Autodesk Fusion 360 part; units mm, degrees
(part 3 of 7)
  spline S363 degree 3 poles (9.5018, -1.5566) (9.5018, -1.7848) (9.4886, -1.9954) (9.4755, -2.0349) knots 0 0 0 0 1 1 1 1
  spline S364 degree 3 poles (9.4755, -2.0349) (9.4404, -2.1271) (9.3701, -2.1227) (9.3701, -2.0305) knots 0 0 0 0 1 1 1 1
  spline S365 degree 3 poles (9.3701, -2.0305) (9.3701, -1.8989) (9.1902, -1.6444) (8.8699, -1.3152) knots 0 0 0 0 1 1 1 1
  spline S366 degree 3 poles (8.8699, -1.3152) (8.7031, -1.1485) (8.5539, -1.008) (8.5407, -1.008) knots 0 0 0 0 1 1 1 1
  spline S367 degree 3 poles (8.5407, -1.008) (8.4925, -1.008) (7.7201, -1.8067) (7.4173, -2.171) knots 0 0 0 0 1 1 1 1
  spline S368 degree 3 poles (7.4173, -2.171) (6.9653, -2.7195) (6.5264, -3.6894) (6.3158, -4.6153) knots 0 0 0 0 1 1 1 1
  spline S369 degree 3 poles (6.3158, -4.6153) (6.1446, -5.3745) (6.1841, -6.1469) (6.4431, -7.0509) knots 0 0 0 0 1 1 1 1
  spline S370 degree 3 poles (6.4431, -7.0509) (6.5923, -7.5731) (6.9302, -8.1392) (7.3646, -8.5913) knots 0 0 0 0 1 1 1 1
  spline S371 degree 3 poles (7.3646, -8.5913) (7.5358, -8.7624) (7.6543, -8.9072) (7.6367, -8.9072) knots 0 0 0 0 1 1 1 1
  spline S372 degree 3 poles (7.6367, -8.9072) (7.5446, -8.9072) (7.2286, -8.6395) (7.0004, -8.3674) knots 0 0 0 0 1 1 1 1
  spline S373 degree 3 poles (7.0004, -8.3674) (6.5791, -7.8672) (6.3114, -7.2659) (6.1183, -6.3839) knots 0 0 0 0 1 1 1 1
  spline S374 degree 3 poles (6.1183, -6.3839) (6.0569, -6.0942) (5.9779, -5.8748) (5.8638, -5.6817) knots 0 0 0 0 1 1 1 1
  spline S375 degree 3 poles (5.8638, -5.6817) (5.776, -5.5237) (5.6882, -5.4052) (5.6795, -5.414) knots 0 0 0 0 1 1 1 1
  spline S376 degree 3 poles (5.6795, -5.414) (5.6487, -5.4491) (5.6312, -5.278) (5.6312, -4.8699) knots 0 0 0 0 1 1 1 1
  spline S377 degree 3 poles (5.6312, -4.8699) (5.6268, -4.5407) (5.6444, -4.453) (5.7892, -4.1019) knots 0 0 0 0 1 1 1 1
  spline S378 degree 3 poles (5.7892, -4.1019) (5.9954, -3.5928) (6.3377, -2.9872) (6.7283, -2.4299) knots 0 0 0 0 1 1 1 1
  spline S379 degree 3 poles (6.7283, -2.4299) (7.0355, -1.991) (7.8254, -1.1441) (8.2511, -0.7974) knots 0 0 0 0 1 1 1 1
  spline S380 degree 3 poles (8.2511, -0.7974) (8.3696, -0.6965) (8.453, -0.6043) (8.4398, -0.5867) knots 0 0 0 0 1 1 1 1
  spline S381 degree 3 poles (8.4398, -0.5867) (8.4047, -0.5516) (7.7201, -0.5516) (7.5709, -0.5867) knots 0 0 0 0 1 1 1 1
  spline S382 degree 3 poles (7.5709, -0.5867) (7.448, -0.6131) (7.3602, -0.714) (7.3207, -0.8676) knots 0 0 0 0 1 1 1 1
  spline S383 degree 3 poles (7.3207, -0.8676) (7.2593, -1.1221) (7.2198, -0.9027) (7.2198, -0.2796) knots 0 0 0 0 1 1 1 1
  spline S384 degree 3 poles (7.2198, -0.2796) (7.2198, 0.3612) (7.2593, 0.5411) (7.3295, 0.2251) knots 0 0 0 0 1 1 1 1
  spline S385 degree 3 poles (7.3295, 0.2251) (7.3427, 0.1549) (7.4085, 0.0452) (7.4699, -0.0163) knots 0 0 0 0 1 1 1 1
  spline S386 degree 3 poles (7.4699, -0.0163) (7.5709, -0.1172) (7.6411, -0.1435) (7.8561, -0.1435) knots 0 0 0 0 1 1 1 1
  spline S387 degree 3 poles (7.8561, -0.1435) (7.8912, -0.1435) (8.4968, -0.1391) (9.2034, -0.1347) knots 0 0 0 0 1 1 1 1
  spline S388 degree 3 poles (9.2034, -0.1347) (10.6998, -0.1304) (10.6603, -0.1567) (9.8353, 0.3392) knots 0 0 0 0 1 1 1 1
  spline S389 degree 3 poles (9.8353, 0.3392) (9.2473, 0.6947) (7.1496, 2.0814) (7.0136, 2.2043) knots 0 0 0 0 1 1 1 1
  spline S390 degree 3 poles (7.0136, 2.2043) (6.9609, 2.2526) (6.8995, 2.2789) (6.8731, 2.2613) knots 0 0 0 0 1 1 1 1
  spline S391 degree 3 poles (6.8731, 2.2613) (6.838, 2.2438) (6.8249, 1.7084) (6.8249, 0.5762) knots 0 0 0 0 1 1 1 1
  spline S392 degree 3 poles (6.8249, 0.5762) (6.8249, -0.3366) (6.8117, -1.2626) (6.7985, -1.482) knots 0 0 0 0 1 1 1 1
  spline S393 degree 3 poles (6.7985, -1.482) (6.7722, -1.8462) (6.759, -1.8901) (6.6581, -1.9559) knots 0 0 0 0 1 1 1 1
  spline S394 degree 3 poles (6.6581, -1.9559) (6.5923, -1.9998) (6.5352, -2.0086) (6.5133, -1.9867) knots 0 0 0 0 1 1 1 1
  spline S395 degree 3 poles (6.5133, -1.9867) (6.4782, -1.9516) (6.4299, 3.0732) (6.465, 3.0732) knots 0 0 0 0 1 1 1 1
  spline S396 degree 3 poles (6.465, 3.0732) (6.4694, 3.0732) (6.5133, 3.0381) (6.5572, 2.9942) knots 0 0 0 0 1 1 1 1
  spline S397 degree 3 poles (6.5572, 2.9942) (6.6405, 2.9196) (7.0399, 2.6475) (8.431, 1.7216) knots 0 0 0 0 1 1 1 1
  spline S398 degree 3 poles (8.431, 1.7216) (8.8172, 1.4627) (9.2824, 1.1511) (9.4623, 1.0282) knots 0 0 0 0 1 1 1 1
  spline S399 degree 3 poles (9.4623, 1.0282) (9.7827, 0.8088) (10.3707, 0.4401) (10.4058, 0.4401) knots 0 0 0 0 1 1 1 1
  spline S400 degree 3 poles (10.4058, 0.4401) (10.4146, 0.4401) (10.4234, 0.7298) (10.4234, 1.0852) knots 0 0 0 0 1 1 1 1
  line L93 (10.4234, 1.0852) -> (10.419, 1.7347)
  line L94 (10.419, 1.7347) -> (10.1732, 1.8839)
  spline S401 degree 3 poles (10.1732, 1.8839) (9.9406, 2.0244) (9.9319, 2.0375) (10.0196, 2.077) knots 0 0 0 0 1 1 1 1
  spline S402 degree 3 poles (10.0196, 2.077) (10.0898, 2.1078) (10.1864, 2.0946) (10.3883, 2.02) knots 0 0 0 0 1 1 1 1
  spline S403 degree 3 poles (10.3883, 2.02) (10.5419, 1.9673) (10.6911, 1.9015) (10.7218, 1.8752) knots 0 0 0 0 1 1 1 1
  spline S404 degree 3 poles (10.7218, 1.8752) (10.7613, 1.8444) (10.7744, 1.6119) (10.7701, 0.9185) knots 0 0 0 0 1 1 1 1
  line L95 (10.7701, 0.9185) -> (10.7657, 0.0013)
  line L96 (10.7657, 0.0013) -> (10.6384, 0.0013)
  spline S405 degree 3 poles (10.6384, 0.0013) (10.5682, 0.0013) (10.5111, -0.0075) (10.5111, -0.0163) knots 0 0 0 0 1 1 1 1
  spline S406 degree 3 poles (10.5111, -0.0163) (10.5111, -0.0514) (10.8798, -0.3849) (11.1475, -0.5955) knots 0 0 0 0 1 1 1 1
  spline S407 degree 3 poles (11.1475, -0.5955) (11.5863, -0.9378) (12.0032, -1.3679) (12.0032, -1.482) knots 0 0 0 0 1 1 1 1
  spline S408 degree 3 poles (12.0032, -1.482) (12.0032, -1.5698) (11.9593, -1.5478) (11.6214, -1.2889) knots 0 0 0 0 1 1 1 1
  spline S409 degree 3 poles (11.2089, 5.9652) (11.1343, 5.9257) (11.1255, 5.9432) (11.1255, 6.1319) knots 0 0 0 0 1 1 1 1
  spline S410 degree 3 poles (11.1255, 6.1319) (11.1255, 6.404) (11.086, 6.5401) (11.0114, 6.5401) knots 0 0 0 0 1 1 1 1
  spline S411 degree 3 poles (11.0114, 6.5401) (10.9763, 6.5401) (10.8008, 6.4699) (10.6165, 6.3865) knots 0 0 0 0 1 1 1 1
  spline S412 degree 3 poles (10.6165, 6.3865) (10.4365, 6.3031) (10.2698, 6.2329) (10.2522, 6.2329) knots 0 0 0 0 1 1 1 1
  spline S413 degree 3 poles (10.2522, 6.2329) (10.2303, 6.2329) (10.0635, 6.1539) (9.8792, 6.0573) knots 0 0 0 0 1 1 1 1
  spline S414 degree 3 poles (9.8792, 6.0573) (9.6949, 5.9608) (9.5062, 5.8818) (9.4623, 5.8818) knots 0 0 0 0 1 1 1 1
  spline S415 degree 3 poles (9.4623, 5.8818) (9.414, 5.8818) (9.3658, 5.8643) (9.3482, 5.8423) knots 0 0 0 0 1 1 1 1
  spline S416 degree 3 poles (9.3482, 5.8423) (9.335, 5.8204) (9.1639, 5.737) (8.9664, 5.6624) knots 0 0 0 0 1 1 1 1
  spline S417 degree 3 poles (8.9664, 5.6624) (8.4661, 5.4693) (8.0799, 5.2674) (8.1238, 5.2235) knots 0 0 0 0 1 1 1 1
  spline S418 degree 3 poles (8.1238, 5.2235) (8.1458, 5.206) (8.2335, 5.1665) (8.3169, 5.1445) knots 0 0 0 0 1 1 1 1
  spline S419 degree 3 poles (8.3169, 5.1445) (8.4003, 5.1182) (8.7163, 5.0041) (9.0191, 4.89) knots 0 0 0 0 1 1 1 1
  spline S420 degree 3 poles (9.0191, 4.89) (9.3394, 4.7671) (9.6422, 4.6794) (9.7432, 4.6794) knots 0 0 0 0 1 1 1 1
  spline S421 degree 3 poles (9.7432, 4.6794) (9.9055, 4.6794) (10.8842, 5.0348) (11.029, 5.1489) knots 0 0 0 0 1 1 1 1
  spline S422 degree 3 poles (11.029, 5.1489) (11.0553, 5.1709) (11.0816, 5.2762) (11.0816, 5.3771) knots 0 0 0 0 1 1 1 1
  spline S423 degree 3 poles (11.0816, 5.3771) (11.0816, 5.5702) (11.1694, 5.6975) (11.2616, 5.6361) knots 0 0 0 0 1 1 1 1
  spline S424 degree 3 poles (11.2616, 5.6361) (11.3318, 5.5966) (11.2923, 3.8807) (11.2221, 3.8105) knots 0 0 0 0 1 1 1 1
  spline S425 degree 3 poles (11.2221, 3.8105) (11.1431, 3.7315) (11.0816, 3.9597) (11.0816, 4.3064) knots 0 0 0 0 1 1 1 1
  spline S426 degree 3 poles (11.0816, 4.3064) (11.0816, 4.7189) (11.1299, 4.7233) (9.9406, 4.2361) knots 0 0 0 0 1 1 1 1
  spline S427 degree 3 poles (9.9406, 4.2361) (9.6861, 4.1352) (9.2385, 3.9553) (8.9445, 3.8412) knots 0 0 0 0 1 1 1 1
  spline S428 degree 3 poles (8.9445, 3.8412) (8.6504, 3.7271) (8.374, 3.6086) (8.3301, 3.5779) knots 0 0 0 0 1 1 1 1
  spline S429 degree 3 poles (8.3301, 3.5779) (8.2599, 3.5252) (8.2686, 3.512) (8.4486, 3.4287) knots 0 0 0 0 1 1 1 1
  spline S430 degree 3 poles (8.4486, 3.4287) (8.9532, 3.2005) (10.8578, 2.4588) (10.95, 2.4588) knots 0 0 0 0 1 1 1 1
  spline S431 degree 3 poles (10.95, 2.4588) (11.007, 2.4588) (11.1255, 2.7441) (11.1255, 2.8845) knots 0 0 0 0 1 1 1 1
  spline S432 degree 3 poles (11.1255, 2.8845) (11.1255, 2.9503) (11.1475, 3.0381) (11.1694, 3.0732) knots 0 0 0 0 1 1 1 1
  spline S433 degree 3 poles (11.1694, 3.0732) (11.2659, 3.218) (11.2967, 2.9898) (11.2967, 2.1516) knots 0 0 0 0 1 1 1 1
  spline S434 degree 3 poles (11.2967, 2.1516) (11.2967, 1.4978) (11.2835, 1.2783) (11.2396, 1.2169) knots 0 0 0 0 1 1 1 1
  spline S435 degree 3 poles (11.2396, 1.2169) (11.1606, 1.1116) (11.1431, 1.1511) (11.1036, 1.5153) knots 0 0 0 0 1 1 1 1
  spline S436 degree 3 poles (11.1036, 1.5153) (11.0553, 2.0112) (11.0641, 1.998) (10.7174, 2.1429) knots 0 0 0 0 1 1 1 1
  spline S437 degree 3 poles (10.7174, 2.1429) (8.6812, 2.981) (7.3032, 3.512) (7.1584, 3.512) knots 0 0 0 0 1 1 1 1
  spline S438 degree 3 poles (7.1584, 3.512) (7.1189, 3.512) (7.0882, 3.5296) (7.0882, 3.5559) knots 0 0 0 0 1 1 1 1
  spline S439 degree 3 poles (7.0882, 3.5559) (7.0882, 3.6569) (7.29, 3.7402) (8.7294, 4.2361) knots 0 0 0 0 1 1 1 1
  spline S440 degree 3 poles (8.7294, 4.2361) (9.1288, 4.3722) (9.2868, 4.4512) (9.2341, 4.4907) knots 0 0 0 0 1 1 1 1
  spline S441 degree 3 poles (9.2341, 4.4907) (9.2034, 4.517) (8.1063, 4.9163) (7.5358, 5.1138) knots 0 0 0 0 1 1 1 1
  spline S442 degree 3 poles (7.5358, 5.1138) (7.2418, 5.2148) (6.9872, 5.3069) (6.9741, 5.3201) knots 0 0 0 0 1 1 1 1
  spline S443 degree 3 poles (6.9741, 5.3201) (6.9653, 5.3332) (7.1671, 5.4254) (7.4261, 5.522) knots 0 0 0 0 1 1 1 1
  spline S444 degree 3 poles (7.4261, 5.522) (7.9395, 5.7194) (8.4091, 5.9125) (9.5896, 6.4216) knots 0 0 0 0 1 1 1 1
  spline S445 degree 3 poles (9.5896, 6.4216) (10.6033, 6.856) (10.9324, 7.014) (10.9983, 7.0974) knots 0 0 0 0 1 1 1 1
  spline S446 degree 3 poles (10.9983, 7.0974) (11.029, 7.1325) (11.0685, 7.3124) (11.0816, 7.4967) knots 0 0 0 0 1 1 1 1
  spline S447 degree 3 poles (11.0816, 7.4967) (11.0992, 7.7688) (11.1167, 7.8347) (11.1782, 7.8478) knots 0 0 0 0 1 1 1 1
  spline S448 degree 3 poles (11.1782, 7.8478) (11.2484, 7.861) (11.2572, 7.8039) (11.2703, 7.2993) knots 0 0 0 0 1 1 1 1
  spline S449 degree 3 poles (11.2703, 7.2993) (11.3011, 6.1012) (11.2967, 6.0135) (11.2089, 5.9652) knots 0 0 0 0 1 1 1 1
  spline S450 degree 3 poles (9.4799, -5.2648) (9.3701, -5.2648) (9.2824, -5.278) (9.2824, -5.2911) knots 0 0 0 0 1 1 1 1
  spline S451 degree 3 poles (9.2824, -5.2911) (9.2824, -5.3087) (9.3614, -5.436) (9.4579, -5.5808) knots 0 0 0 0 1 1 1 1
  spline S452 degree 3 poles (9.4579, -5.5808) (9.6071, -5.8046) (9.6334, -5.8792) (9.6334, -6.0723) knots 0 0 0 0 1 1 1 1
  spline S453 degree 3 poles (9.6334, -6.0723) (9.6291, -6.476) (9.4052, -6.8139) (9.0761, -6.8929) knots 0 0 0 0 1 1 1 1
  spline S454 degree 3 poles (9.0761, -6.8929) (8.984, -6.9149) (8.6548, -6.9324) (8.3389, -6.9368) knots 0 0 0 0 1 1 1 1
  spline S455 degree 3 poles (8.3389, -6.9368) (8.0273, -6.9368) (7.6806, -6.9631) (7.5709, -6.9895) knots 0 0 0 0 1 1 1 1
  spline S456 degree 3 poles (7.5709, -6.9895) (7.3866, -7.0377) (7.369, -7.0553) (7.2988, -7.2616) knots 0 0 0 0 1 1 1 1
  line L97 (7.2988, -7.2616) -> (7.2242, -7.481)
  line L98 (7.2242, -7.481) -> (7.2242, -6.8227)
  spline S457 degree 3 poles (7.2242, -6.8227) (7.2242, -6.2171) (7.2286, -6.1732) (7.29, -6.2829) knots 0 0 0 0 1 1 1 1
  spline S458 degree 3 poles (7.29, -6.2829) (7.4041, -6.498) (7.5489, -6.5375) (8.2379, -6.5462) knots 0 0 0 0 1 1 1 1
  spline S459 degree 3 poles (8.2379, -6.5462) (8.9225, -6.555) (9.0498, -6.5243) (9.2034, -6.3137) knots 0 0 0 0 1 1 1 1
  spline S460 degree 3 poles (9.2034, -6.3137) (9.3745, -6.0811) (9.357, -5.5983) (9.1727, -5.414) knots 0 0 0 0 1 1 1 1
  spline S461 degree 3 poles (9.1727, -5.414) (9.0717, -5.3131) (9.0454, -5.3087) (8.4135, -5.3087) knots 0 0 0 0 1 1 1 1
  spline S462 degree 3 poles (8.4135, -5.3087) (8.0536, -5.3087) (7.6981, -5.3306) (7.6235, -5.357) knots 0 0 0 0 1 1 1 1
  spline S463 degree 3 poles (7.6235, -5.357) (7.4831, -5.4052) (7.3076, -5.6334) (7.3076, -5.7651) knots 0 0 0 0 1 1 1 1
  spline S464 degree 3 poles (7.3076, -5.7651) (7.3076, -5.8046) (7.2812, -5.8353) (7.2549, -5.8353) knots 0 0 0 0 1 1 1 1
  spline S465 degree 3 poles (7.2549, -5.8353) (7.211, -5.8353) (7.1979, -5.6773) (7.1979, -5.1814) knots 0 0 0 0 1 1 1 1
  spline S466 degree 3 poles (7.1979, -5.1814) (7.1979, -4.51) (7.233, -4.4047) (7.3559, -4.7031) knots 0 0 0 0 1 1 1 1
  spline S467 degree 3 poles (7.3559, -4.7031) (7.3866, -4.7733) (7.4568, -4.8523) (7.5138, -4.8742) knots 0 0 0 0 1 1 1 1
  spline S468 degree 3 poles (7.5138, -4.8742) (7.6323, -4.9181) (8.8874, -4.9269) (9.1024, -4.8874) knots 0 0 0 0 1 1 1 1
  spline S469 degree 3 poles (9.1024, -4.8874) (9.1902, -4.8699) (9.2385, -4.8348) (9.2385, -4.7821) knots 0 0 0 0 1 1 1 1
  spline S470 degree 3 poles (9.2385, -4.7821) (9.2385, -4.7426) (9.278, -4.6724) (9.3219, -4.6329) knots 0 0 0 0 1 1 1 1
  spline S471 degree 3 poles (9.3219, -4.6329) (9.414, -4.5495) (9.4184, -4.5495) (9.4799, -4.8523) knots 0 0 0 0 1 1 1 1
  spline S472 degree 3 poles (9.4799, -4.8523) (9.493, -4.9313) (9.5457, -5.0278) (9.594, -5.0717) knots 0 0 0 0 1 1 1 1
  spline S473 degree 3 poles (9.594, -5.0717) (9.7344, -5.199) (9.6993, -5.2648) (9.4799, -5.2648) knots 0 0 0 0 1 1 1 1
  spline S474 degree 3 poles (9.5369, -3.7376) (9.4755, -3.9483) (9.2078, -4.1984) (9.0015, -4.2379) knots 0 0 0 0 1 1 1 1
  spline S475 degree 3 poles (9.0015, -4.2379) (8.7119, -4.2906) (8.7163, -4.295) (8.7031, -3.4787) knots 0 0 0 0 1 1 1 1
  line L99 (8.7031, -3.4787) -> (8.6899, -2.7415)
  line L100 (8.6899, -2.7415) -> (8.352, -2.7415)
  spline S476 degree 3 poles (8.352, -2.7415) (8.0448, -2.7415) (8.0053, -2.7502) (7.8517, -2.8775) knots 0 0 0 0 1 1 1 1
  spline S477 degree 3 poles (7.8517, -2.8775) (7.5007, -3.1584) (7.4085, -3.5928) (7.6279, -3.9527) knots 0 0 0 0 1 1 1 1
  spline S478 degree 3 poles (7.6279, -3.9527) (7.6938, -4.058) (7.7947, -4.2072) (7.8605, -4.2862) knots 0 0 0 0 1 1 1 1
  spline S479 degree 3 poles (7.8605, -4.2862) (8.0185, -4.4793) (7.9307, -4.4968) (7.6718, -4.3213) knots 0 0 0 0 1 1 1 1
  spline S480 degree 3 poles (7.6718, -4.3213) (6.9477, -3.8342) (6.9697, -2.8863) (7.7113, -2.4738) knots 0 0 0 0 1 1 1 1
  spline S481 degree 3 poles (7.7113, -2.4738) (7.9176, -2.3597) (7.9878, -2.3465) (8.3389, -2.3465) knots 0 0 0 0 1 1 1 1
  spline S482 degree 3 poles (8.3389, -2.3465) (8.8304, -2.3465) (8.9137, -2.3685) (9.1858, -2.5835) knots 0 0 0 0 1 1 1 1
  spline S483 degree 3 poles (9.1858, -2.5835) (9.5501, -2.8731) (9.6729, -3.2812) (9.5369, -3.7376) knots 0 0 0 0 1 1 1 1
  spline S484 degree 3 poles (9.3263, -2.996) (9.2912, -2.9038) (9.0761, -2.7634) (8.9752, -2.7634) knots 0 0 0 0 1 1 1 1
  spline S485 degree 3 poles (8.9752, -2.7634) (8.9225, -2.7634) (8.9137, -3.7991) (8.9664, -3.8342) knots 0 0 0 0 1 1 1 1
  spline S486 degree 3 poles (8.9664, -3.8342) (9.0191, -3.8649) (9.2692, -3.6016) (9.3219, -3.4524) knots 0 0 0 0 1 1 1 1
  spline S487 degree 3 poles (9.3219, -3.4524) (9.3789, -3.3076) (9.3789, -3.1277) (9.3263, -2.996) knots 0 0 0 0 1 1 1 1
extrude "拉伸6" cut sketch "草图4" against normal blind 1 contours S227 S228 S229 S230 S231 S232 S233 S234 S235 S236 L69 L70 S237 S238 S239 S240 S241 S242 S243 S244 S245 L71 L72 S246 S247 S248 S249 S250 S251 S252 S253 S254 | S255 S256 S257 S258 S259 S260 S261 S262 S263 S264 S265 S266 S267 S268 S269 S270 S271 S272 S273 | S274 S275 S276 S277 S278 S279 S280 S281 S282 S283 S284 S285 S286 S287 S288 L73 L74 S289 S290 S291 S292 S293 L75 L76 S294 S295 S296 S297 S298 S299 S300 S301 S302 S303 S304 S305 S306 S307 S308 S309 S310 S311 S312 S313 S314 S315 S316 | S317 S318 S319 S320 S321 S322 S323 L77 L78 S324 S325 S326 S327 S328 S329 S330 S331 S332 S333 S334 S335 S336 S337 | S338 S339 S340 S341 S342 S343 S344 S345 S346 S347 L79 L80 S348 S349 S350 | S357 S358 L89 L90 S359 S360 L91 L92 S361 S362 S363 S364 S365 S366 S367 S368 S369 S370 S371 S372 S373 S374 S375 S376 S377 S378 S379 S380 S381 S382 S383 S384 S385 S386 S387 S388 S389 S390 S391 S392 S393 S394 S395 S396 S397 S398 S399 S400 L93 L94 S401 S402 S403 S404 L95 L96 S405 S406 S407 S408 | S409 S410 S411 S412 S413 S414 S415 S416 S417 S418 S419 S420 S421 S422 S423 S424 S425 S426 S427 S428 S429 S430 S431 S432 S433 S434 S435 S436 S437 S438 S439 S440 S441 S442 S443 S444 S445 S446 S447 S448 S449 | S450 S451 S452 S453 S454 S455 S456 L97 L98 S457 S458 S459 S460 S461 S462 S463 S464 S465 S466 S467 S468 S469 S470 S471 S472 S473 | S474 S475 L99 L100 S476 S477 S478 S479 S480 S481 S482 S483
sketch "草图5" plane through (0, 2, 0) normal (0, 1, 0) x (-1, 0, 0)
  spline S0 degree 3 poles (-8.2499, -0.5247) (-8.9348, -0.374) (-9.2773, -0.2416) (-9.9851, 0.1602) knots 0 0 0 0 1 1 1 1
  spline S1 degree 3 poles (-9.9851, 0.1602) (-10.7249, 0.5804) (-11.2318, 0.9959) (-11.5286, 1.4252) knots 0 0 0 0 1 1 1 1
  spline S2 degree 3 poles (-11.5286, 1.4252) (-11.7843, 1.7905) (-11.8254, 2.0188) (-11.6839, 2.3019) knots 0 0 0 0 1 1 1 1
  spline S3 degree 3 poles (-11.6839, 2.3019) (-11.5971, 2.4663) (-11.4464, 2.5896) (-11.3642, 2.5622) knots 0 0 0 0 1 1 1 1
  spline S4 degree 3 poles (-11.3642, 2.5622) (-11.2775, 2.5257) (-11.2775, 2.4207) (-11.3597, 2.3476) knots 0 0 0 0 1 1 1 1
  spline S5 degree 3 poles (-11.3597, 2.3476) (-11.3962, 2.3202) (-11.4601, 2.206) (-11.5012, 2.101) knots 0 0 0 0 1 1 1 1
  spline S6 degree 3 poles (-11.5012, 2.101) (-11.5606, 1.9549) (-11.5652, 1.8818) (-11.5241, 1.7813) knots 0 0 0 0 1 1 1 1
  spline S7 degree 3 poles (-11.5241, 1.7813) (-11.3551, 1.3293) (-9.7568, 0.2607) (-8.8526, -0.0087) knots 0 0 0 0 1 1 1 1
  spline S8 degree 3 poles (-8.8526, -0.0087) (-8.3229, -0.164) (-8.2362, -0.1823) (-8.2362, -0.1412) knots 0 0 0 0 1 1 1 1
  spline S9 degree 3 poles (-8.2362, -0.1412) (-8.2362, -0.0955) (-8.5695, 0.3475) (-8.775, 0.5758) knots 0 0 0 0 1 1 1 1
  spline S10 degree 3 poles (-8.775, 0.5758) (-8.8846, 0.6945) (-8.9714, 0.7493) (-9.0581, 0.7493) knots 0 0 0 0 1 1 1 1
  spline S11 degree 3 poles (-9.0581, 0.7493) (-9.2225, 0.7493) (-9.3687, 0.9091) (-9.3047, 1.0142) knots 0 0 0 0 1 1 1 1
  spline S12 degree 3 poles (-9.3047, 1.0142) (-9.2773, 1.0553) (-9.1997, 1.0964) (-9.1312, 1.1055) knots 0 0 0 0 1 1 1 1
  spline S13 degree 3 poles (-9.1312, 1.1055) (-9.0307, 1.1192) (-8.9577, 1.0644) (-8.7294, 0.8178) knots 0 0 0 0 1 1 1 1
  spline S14 degree 3 poles (-8.7294, 0.8178) (-8.4051, 0.4708) (-8.3092, 0.3292) (-8.2316, 0.0735) knots 0 0 0 0 1 1 1 1
  spline S15 degree 3 poles (-8.2316, 0.0735) (-8.1768, -0.1183) (-8.1311, -0.1457) (-7.5284, -0.3786) knots 0 0 0 0 1 1 1 1
  spline S16 degree 3 poles (-7.5284, -0.3786) (-7.3183, -0.4562) (-7.3, -0.4745) (-7.3137, -0.5978) knots 0 0 0 0 1 1 1 1
  spline S17 degree 3 poles (-7.3137, -0.5978) (-7.3366, -0.7713) (-7.332, -0.7668) (-7.4781, -0.712) knots 0 0 0 0 1 1 1 1
  spline S18 degree 3 poles (-7.4781, -0.712) (-7.5466, -0.6891) (-7.8937, -0.6024) (-8.2499, -0.5247) knots 0 0 0 0 1 1 1 1
  spline S19 degree 3 poles (11.0816, 7.4967) (11.0992, 7.7688) (11.1167, 7.8347) (11.1782, 7.8478) knots 0 0 0 0 1 1 1 1
  spline S20 degree 3 poles (11.1782, 7.8478) (11.2484, 7.861) (11.2572, 7.8039) (11.2703, 7.2993) knots 0 0 0 0 1 1 1 1
  spline S21 degree 3 poles (11.2703, 7.2993) (11.3011, 6.1012) (11.2967, 6.0135) (11.2089, 5.9652) knots 0 0 0 0 1 1 1 1
  spline S22 degree 3 poles (11.2089, 5.9652) (11.1343, 5.9257) (11.1255, 5.9432) (11.1255, 6.1319) knots 0 0 0 0 1 1 1 1
  spline S23 degree 3 poles (11.1255, 6.1319) (11.1255, 6.404) (11.086, 6.5401) (11.0114, 6.5401) knots 0 0 0 0 1 1 1 1
  spline S24 degree 3 poles (11.0114, 6.5401) (10.9763, 6.5401) (10.8008, 6.4699) (10.6165, 6.3865) knots 0 0 0 0 1 1 1 1
  spline S25 degree 3 poles (10.6165, 6.3865) (10.4365, 6.3031) (10.2698, 6.2329) (10.2522, 6.2329) knots 0 0 0 0 1 1 1 1
  spline S26 degree 3 poles (10.2522, 6.2329) (10.2303, 6.2329) (10.0635, 6.1539) (9.8792, 6.0573) knots 0 0 0 0 1 1 1 1
  spline S27 degree 3 poles (9.8792, 6.0573) (9.6949, 5.9608) (9.5062, 5.8818) (9.4623, 5.8818) knots 0 0 0 0 1 1 1 1
  spline S28 degree 3 poles (9.4623, 5.8818) (9.414, 5.8818) (9.3658, 5.8643) (9.3482, 5.8423) knots 0 0 0 0 1 1 1 1
  spline S29 degree 3 poles (9.3482, 5.8423) (9.335, 5.8204) (9.1639, 5.737) (8.9664, 5.6624) knots 0 0 0 0 1 1 1 1
  spline S30 degree 3 poles (8.9664, 5.6624) (8.4661, 5.4693) (8.0799, 5.2674) (8.1238, 5.2235) knots 0 0 0 0 1 1 1 1
  spline S31 degree 3 poles (8.1238, 5.2235) (8.1458, 5.206) (8.2335, 5.1665) (8.3169, 5.1445) knots 0 0 0 0 1 1 1 1
  spline S32 degree 3 poles (8.3169, 5.1445) (8.4003, 5.1182) (8.7163, 5.0041) (9.0191, 4.89) knots 0 0 0 0 1 1 1 1
  spline S33 degree 3 poles (9.0191, 4.89) (9.3394, 4.7671) (9.6422, 4.6794) (9.7432, 4.6794) knots 0 0 0 0 1 1 1 1
  spline S34 degree 3 poles (9.7432, 4.6794) (9.9055, 4.6794) (10.8842, 5.0348) (11.029, 5.1489) knots 0 0 0 0 1 1 1 1
  spline S35 degree 3 poles (11.029, 5.1489) (11.0553, 5.1709) (11.0816, 5.2762) (11.0816, 5.3771) knots 0 0 0 0 1 1 1 1
  spline S36 degree 3 poles (11.0816, 5.3771) (11.0816, 5.5702) (11.1694, 5.6975) (11.2616, 5.6361) knots 0 0 0 0 1 1 1 1
  spline S37 degree 3 poles (11.2616, 5.6361) (11.3318, 5.5966) (11.2923, 3.8807) (11.2221, 3.8105) knots 0 0 0 0 1 1 1 1
  spline S38 degree 3 poles (11.2221, 3.8105) (11.1431, 3.7315) (11.0816, 3.9597) (11.0816, 4.3064) knots 0 0 0 0 1 1 1 1
  spline S39 degree 3 poles (11.0816, 4.3064) (11.0816, 4.7189) (11.1299, 4.7233) (9.9406, 4.2361) knots 0 0 0 0 1 1 1 1
  spline S40 degree 3 poles (9.9406, 4.2361) (9.6861, 4.1352) (9.2385, 3.9553) (8.9445, 3.8412) knots 0 0 0 0 1 1 1 1
  spline S41 degree 3 poles (8.9445, 3.8412) (8.6504, 3.7271) (8.374, 3.6086) (8.3301, 3.5779) knots 0 0 0 0 1 1 1 1
  spline S42 degree 3 poles (8.3301, 3.5779) (8.2599, 3.5252) (8.2686, 3.512) (8.4486, 3.4287) knots 0 0 0 0 1 1 1 1
  spline S43 degree 3 poles (8.4486, 3.4287) (8.9532, 3.2005) (10.8578, 2.4588) (10.95, 2.4588) knots 0 0 0 0 1 1 1 1
  spline S44 degree 3 poles (10.95, 2.4588) (11.007, 2.4588) (11.1255, 2.7441) (11.1255, 2.8845) knots 0 0 0 0 1 1 1 1
  spline S45 degree 3 poles (11.1255, 2.8845) (11.1255, 2.9503) (11.1475, 3.0381) (11.1694, 3.0732) knots 0 0 0 0 1 1 1 1
  spline S46 degree 3 poles (11.1694, 3.0732) (11.2659, 3.218) (11.2967, 2.9898) (11.2967, 2.1516) knots 0 0 0 0 1 1 1 1
  spline S47 degree 3 poles (11.2967, 2.1516) (11.2967, 1.4978) (11.2835, 1.2783) (11.2396, 1.2169) knots 0 0 0 0 1 1 1 1
  spline S48 degree 3 poles (11.2396, 1.2169) (11.1606, 1.1116) (11.1431, 1.1511) (11.1036, 1.5153) knots 0 0 0 0 1 1 1 1
  spline S49 degree 3 poles (11.1036, 1.5153) (11.0553, 2.0112) (11.0641, 1.998) (10.7174, 2.1429) knots 0 0 0 0 1 1 1 1
  spline S50 degree 3 poles (10.7174, 2.1429) (8.6812, 2.981) (7.3032, 3.512) (7.1584, 3.512) knots 0 0 0 0 1 1 1 1
  spline S51 degree 3 poles (7.1584, 3.512) (7.1189, 3.512) (7.0882, 3.5296) (7.0882, 3.5559) knots 0 0 0 0 1 1 1 1
  spline S52 degree 3 poles (7.0882, 3.5559) (7.0882, 3.6569) (7.29, 3.7402) (8.7294, 4.2361) knots 0 0 0 0 1 1 1 1
  spline S53 degree 3 poles (8.7294, 4.2361) (9.1288, 4.3722) (9.2868, 4.4512) (9.2341, 4.4907) knots 0 0 0 0 1 1 1 1
  spline S54 degree 3 poles (9.2341, 4.4907) (9.2034, 4.517) (8.1063, 4.9163) (7.5358, 5.1138) knots 0 0 0 0 1 1 1 1
  spline S55 degree 3 poles (7.5358, 5.1138) (7.2418, 5.2148) (6.9872, 5.3069) (6.9741, 5.3201) knots 0 0 0 0 1 1 1 1
  spline S56 degree 3 poles (6.9741, 5.3201) (6.9653, 5.3332) (7.1671, 5.4254) (7.4261, 5.522) knots 0 0 0 0 1 1 1 1
  spline S57 degree 3 poles (7.4261, 5.522) (7.9395, 5.7194) (8.4091, 5.9125) (9.5896, 6.4216) knots 0 0 0 0 1 1 1 1
  spline S58 degree 3 poles (9.5896, 6.4216) (10.6033, 6.856) (10.9324, 7.014) (10.9983, 7.0974) knots 0 0 0 0 1 1 1 1
  spline S59 degree 3 poles (10.9983, 7.0974) (11.029, 7.1325) (11.0685, 7.3124) (11.0816, 7.4967) knots 0 0 0 0 1 1 1 1
  spline S60 degree 3 poles (9.3219, -4.6329) (9.414, -4.5495) (9.4184, -4.5495) (9.4799, -4.8523) knots 0 0 0 0 1 1 1 1
  spline S61 degree 3 poles (9.4799, -4.8523) (9.493, -4.9313) (9.5457, -5.0278) (9.594, -5.0717) knots 0 0 0 0 1 1 1 1
  spline S62 degree 3 poles (9.594, -5.0717) (9.7344, -5.199) (9.6993, -5.2648) (9.4799, -5.2648) knots 0 0 0 0 1 1 1 1
  spline S63 degree 3 poles (9.4799, -5.2648) (9.3701, -5.2648) (9.2824, -5.278) (9.2824, -5.2911) knots 0 0 0 0 1 1 1 1
  spline S64 degree 3 poles (9.2824, -5.2911) (9.2824, -5.3087) (9.3614, -5.436) (9.4579, -5.5808) knots 0 0 0 0 1 1 1 1
  spline S65 degree 3 poles (9.4579, -5.5808) (9.6071, -5.8046) (9.6334, -5.8792) (9.6334, -6.0723) knots 0 0 0 0 1 1 1 1
  spline S66 degree 3 poles (9.6334, -6.0723) (9.6291, -6.476) (9.4052, -6.8139) (9.0761, -6.8929) knots 0 0 0 0 1 1 1 1
  spline S67 degree 3 poles (9.0761, -6.8929) (8.984, -6.9149) (8.6548, -6.9324) (8.3389, -6.9368) knots 0 0 0 0 1 1 1 1
  spline S68 degree 3 poles (8.3389, -6.9368) (8.0273, -6.9368) (7.6806, -6.9631) (7.5709, -6.9895) knots 0 0 0 0 1 1 1 1
  spline S69 degree 3 poles (7.5709, -6.9895) (7.3866, -7.0377) (7.369, -7.0553) (7.2988, -7.2616) knots 0 0 0 0 1 1 1 1
  line L0 (7.2988, -7.2616) -> (7.2242, -7.481)
  line L1 (7.2242, -7.481) -> (7.2242, -6.8227)
  spline S70 degree 3 poles (7.2242, -6.8227) (7.2242, -6.2171) (7.2286, -6.1732) (7.29, -6.2829) knots 0 0 0 0 1 1 1 1
  spline S71 degree 3 poles (7.29, -6.2829) (7.4041, -6.498) (7.5489, -6.5375) (8.2379, -6.5462) knots 0 0 0 0 1 1 1 1
  spline S72 degree 3 poles (8.2379, -6.5462) (8.9225, -6.555) (9.0498, -6.5243) (9.2034, -6.3137) knots 0 0 0 0 1 1 1 1
  spline S73 degree 3 poles (9.2034, -6.3137) (9.3745, -6.0811) (9.357, -5.5983) (9.1727, -5.414) knots 0 0 0 0 1 1 1 1
  spline S74 degree 3 poles (9.1727, -5.414) (9.0717, -5.3131) (9.0454, -5.3087) (8.4135, -5.3087) knots 0 0 0 0 1 1 1 1
  spline S75 degree 3 poles (8.4135, -5.3087) (8.0536, -5.3087) (7.6981, -5.3306) (7.6235, -5.357) knots 0 0 0 0 1 1 1 1
  spline S76 degree 3 poles (7.6235, -5.357) (7.4831, -5.4052) (7.3076, -5.6334) (7.3076, -5.7651) knots 0 0 0 0 1 1 1 1
  spline S77 degree 3 poles (7.3076, -5.7651) (7.3076, -5.8046) (7.2812, -5.8353) (7.2549, -5.8353) knots 0 0 0 0 1 1 1 1
  spline S78 degree 3 poles (7.2549, -5.8353) (7.211, -5.8353) (7.1979, -5.6773) (7.1979, -5.1814) knots 0 0 0 0 1 1 1 1
  spline S79 degree 3 poles (7.1979, -5.1814) (7.1979, -4.51) (7.233, -4.4047) (7.3559, -4.7031) knots 0 0 0 0 1 1 1 1
  spline S80 degree 3 poles (7.3559, -4.7031) (7.3866, -4.7733) (7.4568, -4.8523) (7.5138, -4.8742) knots 0 0 0 0 1 1 1 1
  spline S81 degree 3 poles (7.5138, -4.8742) (7.6323, -4.9181) (8.8874, -4.9269) (9.1024, -4.8874) knots 0 0 0 0 1 1 1 1
  spline S82 degree 3 poles (9.1024, -4.8874) (9.1902, -4.8699) (9.2385, -4.8348) (9.2385, -4.7821) knots 0 0 0 0 1 1 1 1
  spline S83 degree 3 poles (9.2385, -4.7821) (9.2385, -4.7426) (9.278, -4.6724) (9.3219, -4.6329) knots 0 0 0 0 1 1 1 1
  spline S84 degree 3 poles (-8.6654, -2.4975) (-8.5513, -2.3605) (-8.5513, -2.3468) (-8.6152, -2.2052) knots 0 0 0 0 1 1 1 1
  spline S85 degree 3 poles (-8.6152, -2.2052) (-9.0216, -1.3467) (-9.2362, -0.849) (-9.2408, -0.7759) knots 0 0 0 0 1 1 1 1
  spline S86 degree 3 poles (-9.2408, -0.7759) (-9.2408, -0.7485) (-9.186, -0.68) (-9.1221, -0.6161) knots 0 0 0 0 1 1 1 1
  spline S87 degree 3 poles (-9.1221, -0.6161) (-9.0079, -0.5065) (-9.0033, -0.5065) (-8.9394, -0.5978) knots 0 0 0 0 1 1 1 1
  spline S88 degree 3 poles (-8.9394, -0.5978) (-8.7522, -0.849) (-8.3686, -1.2645) (-8.1083, -1.4883) knots 0 0 0 0 1 1 1 1
  spline S89 degree 3 poles (-8.1083, -1.4883) (-7.7613, -1.7851) (-7.1311, -2.2646) (-7.0854, -2.2646) knots 0 0 0 0 1 1 1 1
  spline S90 degree 3 poles (-7.0854, -2.2646) (-7.0306, -2.2646) (-7.0397, -1.8125) (-7.0945, -1.6161) knots 0 0 0 0 1 1 1 1
  spline S91 degree 3 poles (-7.0945, -1.6161) (-7.1265, -1.5065) (-7.2087, -1.3969) (-7.3229, -1.3056) knots 0 0 0 0 1 1 1 1
  spline S92 degree 3 poles (-7.3229, -1.3056) (-7.4233, -1.2234) (-7.5055, -1.1412) (-7.5055, -1.1184) knots 0 0 0 0 1 1 1 1
  spline S93 degree 3 poles (-7.5055, -1.1184) (-7.5055, -1.0956) (-7.3685, -1.0773) (-7.1996, -1.0773) knots 0 0 0 0 1 1 1 1
  line L2 (-7.1996, -1.0773) -> (-6.889, -1.0773)
  line L3 (-6.889, -1.0773) -> (-6.8799, -1.7257)
  spline S94 degree 3 poles (-6.8799, -1.7257) (-6.8662, -2.4929) (-6.7977, -2.7532) (-6.5694, -2.9313) knots 0 0 0 0 1 1 1 1
  spline S95 degree 3 poles (-6.5694, -2.9313) (-6.4872, -2.9952) (-6.3411, -3.0592) (-6.2497, -3.0729) knots 0 0 0 0 1 1 1 1
  spline S96 degree 3 poles (-6.2497, -3.0729) (-5.9483, -3.1231) (-5.994, -3.3149) (-6.3091, -3.3149) knots 0 0 0 0 1 1 1 1
  spline S97 degree 3 poles (-6.3091, -3.3149) (-6.4278, -3.3149) (-6.5192, -3.2555) (-6.8114, -2.9815) knots 0 0 0 0 1 1 1 1
  spline S98 degree 3 poles (-6.8114, -2.9815) (-7.0032, -2.7989) (-7.3366, -2.5066) (-7.5512, -2.3331) knots 0 0 0 0 1 1 1 1
  spline S99 degree 3 poles (-7.5512, -2.3331) (-7.7658, -2.1596) (-8.1174, -1.8582) (-8.3366, -1.6572) knots 0 0 0 0 1 1 1 1
  spline S100 degree 3 poles (-8.3366, -1.6572) (-8.5558, -1.4609) (-8.7568, -1.3056) (-8.7796, -1.3148) knots 0 0 0 0 1 1 1 1
  spline S101 degree 3 poles (-8.7796, -1.3148) (-8.8481, -1.3376) (-8.4417, -2.3285) (-8.3092, -2.4609) knots 0 0 0 0 1 1 1 1
  spline S102 degree 3 poles (-8.3092, -2.4609) (-8.1631, -2.6071) (-8.1631, -2.6482) (-8.3001, -2.7349) knots 0 0 0 0 1 1 1 1
  spline S103 degree 3 poles (-8.3001, -2.7349) (-8.3869, -2.7943) (-8.4417, -2.7989) (-8.5741, -2.7623) knots 0 0 0 0 1 1 1 1
  spline S104 degree 3 poles (-8.5741, -2.7623) (-8.7933, -2.703) (-8.807, -2.6619) (-8.6654, -2.4975) knots 0 0 0 0 1 1 1 1
  spline S105 degree 3 poles (-8.6015, 2.9412) (-8.4462, 2.9412) (-8.4554, 2.9504) (-8.8298, 3.1696) knots 0 0 0 0 1 1 1 1
  spline S106 degree 3 poles (-8.8298, 3.1696) (-9.0444, 3.2929) (-9.2499, 3.439) (-9.2956, 3.4892) knots 0 0 0 0 1 1 1 1
  spline S107 degree 3 poles (-9.2956, 3.4892) (-9.3869, 3.6034) (-9.355, 3.7449) (-9.2088, 3.8408) knots 0 0 0 0 1 1 1 1
  spline S108 degree 3 poles (-9.2088, 3.8408) (-9.0901, 3.9185) (-8.6883, 3.9093) (-8.0763, 3.8089) knots 0 0 0 0 1 1 1 1
  spline S109 degree 3 poles (-8.0763, 3.8089) (-7.4233, 3.7038) (-7.0945, 3.7632) (-7.0352, 3.9915) knots 0 0 0 0 1 1 1 1
  spline S110 degree 3 poles (-7.0352, 3.9915) (-7.0169, 4.0692) (-7.0534, 4.1057) (-7.2361, 4.197) knots 0 0 0 0 1 1 1 1
  spline S111 degree 3 poles (-7.2361, 4.197) (-7.3594, 4.261) (-7.4599, 4.334) (-7.4599, 4.3569) knots 0 0 0 0 1 1 1 1
  spline S112 degree 3 poles (-7.4599, 4.3569) (-7.4599, 4.4893) (-6.9119, 4.2975) (-6.8251, 4.1377) knots 0 0 0 0 1 1 1 1
  spline S113 degree 3 poles (-6.8251, 4.1377) (-6.6973, 3.9002) (-6.816, 3.6125) (-7.1082, 3.4618) knots 0 0 0 0 1 1 1 1
  spline S114 degree 3 poles (-7.1082, 3.4618) (-7.332, 3.3477) (-7.8617, 3.334) (-8.4188, 3.4344) knots 0 0 0 0 1 1 1 1
  spline S115 degree 3 poles (-8.4188, 3.4344) (-8.9759, 3.5349) (-9.0855, 3.5212) (-8.9029, 3.3751) knots 0 0 0 0 1 1 1 1
  spline S116 degree 3 poles (-8.9029, 3.3751) (-8.6974, 3.2107) (-7.9576, 2.859) (-7.6562, 2.7768) knots 0 0 0 0 1 1 1 1
  spline S117 degree 3 poles (-7.6562, 2.7768) (-7.3868, 2.7038) (-7.3685, 2.6946) (-7.3685, 2.5668) knots 0 0 0 0 1 1 1 1
  spline S118 degree 3 poles (-7.3685, 2.5668) (-7.3685, 2.4024) (-7.437, 2.375) (-7.7384, 2.4298) knots 0 0 0 0 1 1 1 1
  spline S119 degree 3 poles (-7.7384, 2.4298) (-7.8754, 2.4572) (-7.9896, 2.4709) (-7.9987, 2.4663) knots 0 0 0 0 1 1 1 1
  spline S120 degree 3 poles (-7.9987, 2.4663) (-8.0033, 2.4572) (-7.8937, 2.3659) (-7.7521, 2.2563) knots 0 0 0 0 1 1 1 1
  spline S121 degree 3 poles (-7.7521, 2.2563) (-7.469, 2.0416) (-7.2315, 1.7083) (-7.2315, 1.5211) knots 0 0 0 0 1 1 1 1
  spline S122 degree 3 poles (-7.2315, 1.5211) (-7.2315, 1.4571) (-7.2818, 1.3247) (-7.3457, 1.2334) knots 0 0 0 0 1 1 1 1
  line L4 (-7.3457, 1.2334) -> (-7.4553, 1.069)
  line L5 (-7.4553, 1.069) -> (-7.2726, 1.069)
  spline S123 degree 3 poles (-7.2726, 1.069) (-7.0671, 1.069) (-6.7566, 0.9274) (-6.711, 0.8178) knots 0 0 0 0 1 1 1 1
  spline S124 degree 3 poles (-6.711, 0.8178) (-6.6425, 0.6351) (-6.6836, 0.4662) (-6.8342, 0.3155) knots 0 0 0 0 1 1 1 1
  spline S125 degree 3 poles (-6.8342, 0.3155) (-7.0078, 0.142) (-7.1996, 0.0826) (-7.7019, 0.0506) knots 0 0 0 0 1 1 1 1
  spline S126 degree 3 poles (-7.7019, 0.0506) (-7.9804, 0.0324) (-8.0672, 0.0415) (-8.1266, 0.0963) knots 0 0 0 0 1 1 1 1
  spline S127 degree 3 poles (-8.1266, 0.0963) (-8.1905, 0.1602) (-8.1859, 0.1785) (-8.0946, 0.2744) knots 0 0 0 0 1 1 1 1
  line L6 (-8.0946, 0.2744) -> (-7.9941, 0.384)
  line L7 (-7.9941, 0.384) -> (-8.1129, 0.384)
  spline S128 degree 3 poles (-8.1129, 0.384) (-8.2088, 0.384) (-8.2362, 0.4068) (-8.2362, 0.4799) knots 0 0 0 0 1 1 1 1
  spline S129 degree 3 poles (-8.2362, 0.4799) (-8.2362, 0.6078) (-8.1585, 0.7356) (-8.0489, 0.7995) knots 0 0 0 0 1 1 1 1
  spline S130 degree 3 poles (-8.0489, 0.7995) (-7.8571, 0.9) (-7.6836, 0.5941) (-7.8663, 0.4662) knots 0 0 0 0 1 1 1 1
  spline S131 degree 3 poles (-7.8663, 0.4662) (-7.9393, 0.416) (-7.9028, 0.4068) (-7.5969, 0.3931) knots 0 0 0 0 1 1 1 1
  spline S132 degree 3 poles (-7.5969, 0.3931) (-7.2955, 0.384) (-7.2315, 0.3931) (-7.1219, 0.4799) knots 0 0 0 0 1 1 1 1
  spline S133 degree 3 poles (-7.1219, 0.4799) (-6.9301, 0.6306) (-6.9712, 0.7904) (-7.2544, 0.9411) knots 0 0 0 0 1 1 1 1
  spline S134 degree 3 poles (-7.2544, 0.9411) (-7.4507, 1.0507) (-7.5284, 1.069) (-7.8297, 1.0598) knots 0 0 0 0 1 1 1 1
  spline S135 degree 3 poles (-7.8297, 1.0598) (-8.1494, 1.0553) (-8.1996, 1.0644) (-8.4234, 1.2014) knots 0 0 0 0 1 1 1 1
  spline S136 degree 3 poles (-8.4234, 1.2014) (-8.8481, 1.4617) (-9.0444, 1.6489) (-9.1266, 1.8681) knots 0 0 0 0 1 1 1 1
  spline S137 degree 3 poles (-9.1266, 1.8681) (-9.2043, 2.0645) (-9.2043, 2.0736) (-9.0992, 2.2882) knots 0 0 0 0 1 1 1 1
  spline S138 degree 3 poles (-9.0992, 2.2882) (-8.9759, 2.5348) (-8.8389, 2.5896) (-8.6837, 2.4526) knots 0 0 0 0 1 1 1 1
  spline S139 degree 3 poles (-8.6837, 2.4526) (-8.5467, 2.3339) (-8.2362, 1.8453) (-8.2362, 1.7539) knots 0 0 0 0 1 1 1 1
  spline S140 degree 3 poles (-8.2362, 1.7539) (-8.2362, 1.5804) (-8.0855, 1.4754) (-7.7932, 1.4389) knots 0 0 0 0 1 1 1 1
  spline S141 degree 3 poles (-7.7932, 1.4389) (-7.4553, 1.3978) (-7.3685, 1.4389) (-7.3685, 1.6215) knots 0 0 0 0 1 1 1 1
  spline S142 degree 3 poles (-7.3685, 1.6215) (-7.3685, 1.7311) (-7.4325, 1.8224) (-7.7019, 2.0782) knots 0 0 0 0 1 1 1 1
  spline S143 degree 3 poles (-7.7019, 2.0782) (-7.88, 2.2563) (-8.0809, 2.4252) (-8.1448, 2.4572) knots 0 0 0 0 1 1 1 1
  spline S144 degree 3 poles (-8.1448, 2.4572) (-8.2773, 2.5257) (-8.9714, 2.7038) (-9.1723, 2.722) knots 0 0 0 0 1 1 1 1
  spline S145 degree 3 poles (-9.1723, 2.722) (-9.2773, 2.7312) (-9.3139, 2.7631) (-9.323, 2.8408) knots 0 0 0 0 1 1 1 1
  spline S146 degree 3 poles (-9.323, 2.8408) (-9.3504, 3.0326) (-9.2728, 3.0737) (-9.0033, 3.0052) knots 0 0 0 0 1 1 1 1
  spline S147 degree 3 poles (-9.0033, 3.0052) (-8.8709, 2.9686) (-8.6928, 2.9412) (-8.6015, 2.9412) knots 0 0 0 0 1 1 1 1
  spline S148 degree 3 poles (7.7113, -2.4738) (7.9176, -2.3597) (7.9878, -2.3465) (8.3389, -2.3465) knots 0 0 0 0 1 1 1 1
  spline S149 degree 3 poles (8.3389, -2.3465) (8.8304, -2.3465) (8.9137, -2.3685) (9.1858, -2.5835) knots 0 0 0 0 1 1 1 1
  spline S150 degree 3 poles (9.1858, -2.5835) (9.5501, -2.8731) (9.6729, -3.2812) (9.5369, -3.7376) knots 0 0 0 0 1 1 1 1
  spline S151 degree 3 poles (9.5369, -3.7376) (9.4755, -3.9483) (9.2078, -4.1984) (9.0015, -4.2379) knots 0 0 0 0 1 1 1 1
  spline S152 degree 3 poles (9.0015, -4.2379) (8.7119, -4.2906) (8.7163, -4.295) (8.7031, -3.4787) knots 0 0 0 0 1 1 1 1
  line L8 (8.7031, -3.4787) -> (8.6899, -2.7415)
  line L9 (8.6899, -2.7415) -> (8.352, -2.7415)
  spline S153 degree 3 poles (8.352, -2.7415) (8.0448, -2.7415) (8.0053, -2.7502) (7.8517, -2.8775) knots 0 0 0 0 1 1 1 1
  spline S154 degree 3 poles (7.8517, -2.8775) (7.5007, -3.1584) (7.4085, -3.5928) (7.6279, -3.9527) knots 0 0 0 0 1 1 1 1
  spline S155 degree 3 poles (7.6279, -3.9527) (7.6938, -4.058) (7.7947, -4.2072) (7.8605, -4.2862) knots 0 0 0 0 1 1 1 1
  spline S156 degree 3 poles (7.8605, -4.2862) (8.0185, -4.4793) (7.9307, -4.4968) (7.6718, -4.3213) knots 0 0 0 0 1 1 1 1
  spline S157 degree 3 poles (7.6718, -4.3213) (6.9477, -3.8342) (6.9697, -2.8863) (7.7113, -2.4738) knots 0 0 0 0 1 1 1 1
  spline S158 degree 3 poles (10.5111, -0.0163) (10.5111, -0.0514) (10.8798, -0.3849) (11.1475, -0.5955) knots 0 0 0 0 1 1 1 1
  spline S159 degree 3 poles (11.1475, -0.5955) (11.5863, -0.9378) (12.0032, -1.3679) (12.0032, -1.482) knots 0 0 0 0 1 1 1 1
  spline S160 degree 3 poles (12.0032, -1.482) (12.0032, -1.5698) (11.9593, -1.5478) (11.6214, -1.2889) knots 0 0 0 0 1 1 1 1
  spline S161 degree 3 poles (11.6214, -1.2889) (11.4064, -1.1309) (11.1782, -0.9422) (11.1036, -0.8764) knots 0 0 0 0 1 1 1 1
  spline S162 degree 3 poles (11.1036, -0.8764) (11.0334, -0.8106) (10.8842, -0.7008) (10.7832, -0.6394) knots 0 0 0 0 1 1 1 1
  line L10 (10.7832, -0.6394) -> (10.5901, -0.5209)
  line L11 (10.5901, -0.5209) -> (9.5983, -0.5253)
  spline S163 degree 3 poles (9.5983, -0.5253) (9.0542, -0.5253) (8.5978, -0.5385) (8.589, -0.5473) knots 0 0 0 0 1 1 1 1
  spline S164 degree 3 poles (8.589, -0.5473) (8.5583, -0.578) (8.6855, -0.7579) (8.984, -1.1046) knots 0 0 0 0 1 1 1 1
  line L12 (8.984, -1.1046) -> (9.256, -1.4162)
  line L13 (9.256, -1.4162) -> (9.3175, -1.2318)
  spline S165 degree 3 poles (9.3175, -1.2318) (9.3658, -1.0826) (9.3921, -1.0563) (9.4404, -1.1002) knots 0 0 0 0 1 1 1 1
  spline S166 degree 3 poles (9.4404, -1.1002) (9.4842, -1.1353) (9.5018, -1.2626) (9.5018, -1.5566) knots 0 0 0 0 1 1 1 1
  spline S167 degree 3 poles (9.5018, -1.5566) (9.5018, -1.7848) (9.4886, -1.9954) (9.4755, -2.0349) knots 0 0 0 0 1 1 1 1
  spline S168 degree 3 poles (9.4755, -2.0349) (9.4404, -2.1271) (9.3701, -2.1227) (9.3701, -2.0305) knots 0 0 0 0 1 1 1 1
  spline S169 degree 3 poles (9.3701, -2.0305) (9.3701, -1.8989) (9.1902, -1.6444) (8.8699, -1.3152) knots 0 0 0 0 1 1 1 1
  spline S170 degree 3 poles (8.8699, -1.3152) (8.7031, -1.1485) (8.5539, -1.008) (8.5407, -1.008) knots 0 0 0 0 1 1 1 1
  spline S171 degree 3 poles (8.5407, -1.008) (8.4925, -1.008) (7.7201, -1.8067) (7.4173, -2.171) knots 0 0 0 0 1 1 1 1
  spline S172 degree 3 poles (7.4173, -2.171) (6.9653, -2.7195) (6.5264, -3.6894) (6.3158, -4.6153) knots 0 0 0 0 1 1 1 1
  spline S173 degree 3 poles (6.3158, -4.6153) (6.1446, -5.3745) (6.1841, -6.1469) (6.4431, -7.0509) knots 0 0 0 0 1 1 1 1
  spline S174 degree 3 poles (6.4431, -7.0509) (6.5923, -7.5731) (6.9302, -8.1392) (7.3646, -8.5913) knots 0 0 0 0 1 1 1 1
  spline S175 degree 3 poles (7.3646, -8.5913) (7.5358, -8.7624) (7.6543, -8.9072) (7.6367, -8.9072) knots 0 0 0 0 1 1 1 1
  spline S176 degree 3 poles (7.6367, -8.9072) (7.5446, -8.9072) (7.2286, -8.6395) (7.0004, -8.3674) knots 0 0 0 0 1 1 1 1
  spline S177 degree 3 poles (7.0004, -8.3674) (6.5791, -7.8672) (6.3114, -7.2659) (6.1183, -6.3839) knots 0 0 0 0 1 1 1 1
  spline S178 degree 3 poles (6.1183, -6.3839) (6.0569, -6.0942) (5.9779, -5.8748) (5.8638, -5.6817) knots 0 0 0 0 1 1 1 1
  spline S179 degree 3 poles (5.8638, -5.6817) (5.776, -5.5237) (5.6882, -5.4052) (5.6795, -5.414) knots 0 0 0 0 1 1 1 1
  spline S180 degree 3 poles (5.6795, -5.414) (5.6487, -5.4491) (5.6312, -5.278) (5.6312, -4.8699) knots 0 0 0 0 1 1 1 1
  spline S181 degree 3 poles (5.6312, -4.8699) (5.6268, -4.5407) (5.6444, -4.453) (5.7892, -4.1019) knots 0 0 0 0 1 1 1 1
  spline S182 degree 3 poles (5.7892, -4.1019) (5.9954, -3.5928) (6.3377, -2.9872) (6.7283, -2.4299) knots 0 0 0 0 1 1 1 1
  spline S183 degree 3 poles (6.7283, -2.4299) (7.0355, -1.991) (7.8254, -1.1441) (8.2511, -0.7974) knots 0 0 0 0 1 1 1 1
  spline S184 degree 3 poles (8.2511, -0.7974) (8.3696, -0.6965) (8.453, -0.6043) (8.4398, -0.5867) knots 0 0 0 0 1 1 1 1
  spline S185 degree 3 poles (8.4398, -0.5867) (8.4047, -0.5516) (7.7201, -0.5516) (7.5709, -0.5867) knots 0 0 0 0 1 1 1 1
  spline S186 degree 3 poles (7.5709, -0.5867) (7.448, -0.6131) (7.3602, -0.714) (7.3207, -0.8676) knots 0 0 0 0 1 1 1 1
  spline S187 degree 3 poles (7.3207, -0.8676) (7.2593, -1.1221) (7.2198, -0.9027) (7.2198, -0.2796) knots 0 0 0 0 1 1 1 1
  spline S188 degree 3 poles (7.2198, -0.2796) (7.2198, 0.3612) (7.2593, 0.5411) (7.3295, 0.2251) knots 0 0 0 0 1 1 1 1
  spline S189 degree 3 poles (7.3295, 0.2251) (7.3427, 0.1549) (7.4085, 0.0452) (7.4699, -0.0163) knots 0 0 0 0 1 1 1 1
  spline S190 degree 3 poles (7.4699, -0.0163) (7.5709, -0.1172) (7.6411, -0.1435) (7.8561, -0.1435) knots 0 0 0 0 1 1 1 1
  spline S191 degree 3 poles (7.8561, -0.1435) (7.8912, -0.1435) (8.4968, -0.1391) (9.2034, -0.1347) knots 0 0 0 0 1 1 1 1
  spline S192 degree 3 poles (9.2034, -0.1347) (10.6998, -0.1304) (10.6603, -0.1567) (9.8353, 0.3392) knots 0 0 0 0 1 1 1 1
  spline S193 degree 3 poles (9.8353, 0.3392) (9.2473, 0.6947) (7.1496, 2.0814) (7.0136, 2.2043) knots 0 0 0 0 1 1 1 1
  spline S194 degree 3 poles (7.0136, 2.2043) (6.9609, 2.2526) (6.8995, 2.2789) (6.8731, 2.2613) knots 0 0 0 0 1 1 1 1
  spline S195 degree 3 poles (6.8731, 2.2613) (6.838, 2.2438) (6.8249, 1.7084) (6.8249, 0.5762) knots 0 0 0 0 1 1 1 1
  spline S196 degree 3 poles (6.8249, 0.5762) (6.8249, -0.3366) (6.8117, -1.2626) (6.7985, -1.482) knots 0 0 0 0 1 1 1 1
  spline S197 degree 3 poles (6.7985, -1.482) (6.7722, -1.8462) (6.759, -1.8901) (6.6581, -1.9559) knots 0 0 0 0 1 1 1 1
  spline S198 degree 3 poles (6.6581, -1.9559) (6.5923, -1.9998) (6.5352, -2.0086) (6.5133, -1.9867) knots 0 0 0 0 1 1 1 1
  spline S199 degree 3 poles (6.5133, -1.9867) (6.4782, -1.9516) (6.4299, 3.0732) (6.465, 3.0732) knots 0 0 0 0 1 1 1 1
  spline S200 degree 3 poles (6.465, 3.0732) (6.4694, 3.0732) (6.5133, 3.0381) (6.5572, 2.9942) knots 0 0 0 0 1 1 1 1
  spline S201 degree 3 poles (6.5572, 2.9942) (6.6405, 2.9196) (7.0399, 2.6475) (8.431, 1.7216) knots 0 0 0 0 1 1 1 1
  spline S202 degree 3 poles (8.431, 1.7216) (8.8172, 1.4627) (9.2824, 1.1511) (9.4623, 1.0282) knots 0 0 0 0 1 1 1 1
  spline S203 degree 3 poles (9.4623, 1.0282) (9.7827, 0.8088) (10.3707, 0.4401) (10.4058, 0.4401) knots 0 0 0 0 1 1 1 1
  spline S204 degree 3 poles (10.4058, 0.4401) (10.4146, 0.4401) (10.4234, 0.7298) (10.4234, 1.0852) knots 0 0 0 0 1 1 1 1
  line L14 (10.4234, 1.0852) -> (10.419, 1.7347)
  line L15 (10.419, 1.7347) -> (10.1732, 1.8839)
  spline S205 degree 3 poles (10.1732, 1.8839) (9.9406, 2.0244) (9.9319, 2.0375) (10.0196, 2.077) knots 0 0 0 0 1 1 1 1
  spline S206 degree 3 poles (10.0196, 2.077) (10.0898, 2.1078) (10.1864, 2.0946) (10.3883, 2.02) knots 0 0 0 0 1 1 1 1
  spline S207 degree 3 poles (10.3883, 2.02) (10.5419, 1.9673) (10.6911, 1.9015) (10.7218, 1.8752) knots 0 0 0 0 1 1 1 1
  spline S208 degree 3 poles (10.7218, 1.8752) (10.7613, 1.8444) (10.7744, 1.6119) (10.7701, 0.9185) knots 0 0 0 0 1 1 1 1
  line L16 (10.7701, 0.9185) -> (10.7657, 0.0013)
  line L17 (10.7657, 0.0013) -> (10.6384, 0.0013)
  spline S209 degree 3 poles (10.6384, 0.0013) (10.5682, 0.0013) (10.5111, -0.0075) (10.5111, -0.0163) knots 0 0 0 0 1 1 1 1
  spline S210 degree 3 poles (-9.9714, -3.1094) (-11.1724, -2.8628) (-11.3597, -2.8171) (-11.6565, -2.6756) knots 0 0 0 0 1 1 1 1
  spline S211 degree 3 poles (-11.6565, -2.6756) (-11.9487, -2.534) (-12.2775, -2.2326) (-12.3734, -2.0134) knots 0 0 0 0 1 1 1 1
  spline S212 degree 3 poles (-12.3734, -2.0134) (-12.4556, -1.8262) (-12.4511, -1.575) (-12.3643, -1.4517) knots 0 0 0 0 1 1 1 1
  spline S213 degree 3 poles (-12.3643, -1.4517) (-12.2912, -1.3467) (-12.1451, -1.3193) (-12.0949, -1.3969) knots 0 0 0 0 1 1 1 1
  spline S214 degree 3 poles (-12.0949, -1.3969) (-12.0812, -1.4198) (-12.0994, -1.4883) (-12.136, -1.5431) knots 0 0 0 0 1 1 1 1
  spline S215 degree 3 poles (-12.136, -1.5431) (-12.2456, -1.6983) (-12.2227, -1.8764) (-12.0766, -2.05) knots 0 0 0 0 1 1 1 1
  spline S216 degree 3 poles (-12.0766, -2.05) (-11.8802, -2.2692) (-11.5834, -2.4153) (-10.8391, -2.6436) knots 0 0 0 0 1 1 1 1
  spline S217 degree 3 poles (-10.8391, -2.6436) (-10.1861, -2.8491) (-6.8434, -3.6939) (-6.4644, -3.7533) knots 0 0 0 0 1 1 1 1
  spline S218 degree 3 poles (-6.4644, -3.7533) (-6.3593, -3.7715) (-6.2589, -3.7989) (-6.2497, -3.8172) knots 0 0 0 0 1 1 1 1
  spline S219 degree 3 poles (-6.2497, -3.8172) (-6.1949, -3.904) (-6.5831, -3.9862) (-8.4371, -4.2739) knots 0 0 0 0 1 1 1 1
  spline S220 degree 3 poles (-8.4371, -4.2739) (-8.9074, -4.3469) (-9.3047, -4.4154) (-9.3139, -4.4245) knots 0 0 0 0 1 1 1 1
  spline S221 degree 3 poles (-9.3139, -4.4245) (-9.3321, -4.4428) (-8.6746, -4.6026) (-7.6654, -4.8218) knots 0 0 0 0 1 1 1 1
  spline S222 degree 3 poles (-7.6654, -4.8218) (-7.3411, -4.8949) (-7.0215, -4.9725) (-6.9575, -4.9954) knots 0 0 0 0 1 1 1 1
  line L18 (-6.9575, -4.9954) -> (-6.8434, -5.041)
  line L19 (-6.8434, -5.041) -> (-6.9575, -5.0684)
  spline S223 degree 3 poles (-6.9575, -5.0684) (-7.0215, -5.0821) (-7.3274, -5.1461) (-7.6425, -5.21) knots 0 0 0 0 1 1 1 1
  spline S224 degree 3 poles (-7.6425, -5.21) (-8.3275, -5.3515) (-9.3504, -5.6027) (-9.8801, -5.7671) knots 0 0 0 0 1 1 1 1
  spline S225 degree 3 poles (-9.8801, -5.7671) (-10.8162, -6.0457) (-11.2592, -6.4338) (-11.2592, -6.9681) knots 0 0 0 0 1 1 1 1
  spline S226 degree 3 poles (-11.2592, -6.9681) (-11.2546, -7.475) (-10.8893, -7.7992) (-10.5697, -7.58) knots 0 0 0 0 1 1 1 1
  spline S227 degree 3 poles (-10.5697, -7.58) (-10.4098, -7.4658) (-10.3459, -7.5709) (-10.5012, -7.6942) knots 0 0 0 0 1 1 1 1
  spline S228 degree 3 poles (-10.5012, -7.6942) (-10.7477, -7.886) (-11.1176, -7.7672) (-11.2729, -7.443) knots 0 0 0 0 1 1 1 1
  spline S229 degree 3 poles (-11.2729, -7.443) (-11.3916, -7.1964) (-11.4145, -6.7124) (-11.3231, -6.4338) knots 0 0 0 0 1 1 1 1
  spline S230 degree 3 poles (-11.3231, -6.4338) (-11.0994, -5.7625) (-10.5377, -5.4657) (-8.8526, -5.1415) knots 0 0 0 0 1 1 1 1
  spline S231 degree 3 poles (-8.8526, -5.1415) (-8.5787, -5.0913) (-8.3001, -5.0319) (-8.2362, -5.0182) knots 0 0 0 0 1 1 1 1
  line L20 (-8.2362, -5.0182) -> (-8.122, -4.9954)
  line L21 (-8.122, -4.9954) -> (-8.2362, -4.9497)
  spline S232 degree 3 poles (-8.2362, -4.9497) (-8.428, -4.8766) (-9.9166, -4.4565) (-10.3322, -4.3606) knots 0 0 0 0 1 1 1 1
  spline S233 degree 3 poles (-10.3322, -4.3606) (-11.0628, -4.1917) (-11.0583, -4.1643) (-10.2591, -4.1232) knots 0 0 0 0 1 1 1 1
  spline S234 degree 3 poles (-10.2591, -4.1232) (-9.9395, -4.1049) (-9.2545, -4.0318) (-8.7385, -3.9542) knots 0 0 0 0 1 1 1 1
  spline S235 degree 3 poles (-8.7385, -3.9542) (-8.2225, -3.8811) (-7.711, -3.8172) (-7.5969, -3.8172) knots 0 0 0 0 1 1 1 1
  spline S236 degree 3 poles (-7.5969, -3.8172) (-7.4781, -3.8172) (-7.4142, -3.7989) (-7.437, -3.7761) knots 0 0 0 0 1 1 1 1
  spline S237 degree 3 poles (-7.437, -3.7761) (-7.5512, -3.6711) (-8.6974, -3.3697) (-9.9714, -3.1094) knots 0 0 0 0 1 1 1 1
  spline S238 degree 3 poles (-6.7292, 7.0054) (-7.0352, 7.5534) (-7.4553, 7.3479) (-7.7795, 6.494) knots 0 0 0 0 1 1 1 1
  spline S239 degree 3 poles (-7.7795, 6.494) (-7.9211, 6.1241) (-8.0078, 6.0008) (-8.1311, 6.0008) knots 0 0 0 0 1 1 1 1
  spline S240 degree 3 poles (-8.1311, 6.0008) (-8.2225, 6.0008) (-8.2042, 6.1561) (-8.0535, 6.5396) knots 0 0 0 0 1 1 1 1
  spline S241 degree 3 poles (-8.0535, 6.5396) (-7.8754, 6.9963) (-7.7293, 7.2109) (-7.5055, 7.3251) knots 0 0 0 0 1 1 1 1
  spline S242 degree 3 poles (-7.5055, 7.3251) (-7.0626, 7.5488) (-6.7292, 7.3662) (-6.5466, 6.7999) knots 0 0 0 0 1 1 1 1
  spline S243 degree 3 poles (-6.5466, 6.7999) (-6.4507, 6.494) (-6.4415, 6.3753) (-6.405, 4.2884) knots 0 0 0 0 1 1 1 1
  spline S244 degree 3 poles (-6.405, 4.2884) (-6.3776, 2.4207) (-6.3, 0.8863) (-6.2041, 0.1557) knots 0 0 0 0 1 1 1 1
  spline S245 degree 3 poles (-6.2041, 0.1557) (-5.9392, -1.8125) (-5.6926, -3.1094) (-5.2862, -4.6163) knots 0 0 0 0 1 1 1 1
  spline S246 degree 3 poles (-5.2862, -4.6163) (-5.1446, -5.1415) (-5.0122, -5.6118) (-4.9848, -5.6575) knots 0 0 0 0 1 1 1 1
  spline S247 degree 3 poles (-4.9848, -5.6575) (-4.962, -5.7032) (-4.9528, -5.7534) (-4.962, -5.7671) knots 0 0 0 0 1 1 1 1
  spline S248 degree 3 poles (-4.962, -5.7671) (-5.0122, -5.8173) (-5.4095, -4.8264) (-5.6515, -4.0455) knots 0 0 0 0 1 1 1 1
  spline S249 degree 3 poles (-5.6515, -4.0455) (-5.8387, -3.4336) (-6.236, -1.4928) (-6.3411, -0.6663) knots 0 0 0 0 1 1 1 1
  spline S250 degree 3 poles (-6.3411, -0.6663) (-6.542, 0.9685) (-6.5603, 1.2379) (-6.5877, 4.0372) knots 0 0 0 0 1 1 1 1
  line L22 (-6.5877, 4.0372) -> (-6.6151, 6.7999)
  line L23 (-6.6151, 6.7999) -> (-6.7292, 7.0054)
  spline S251 degree 3 poles (0.4584, 12.176) (0.7918, 12.3856) (1.2919, 12.7285) (1.5681, 12.9333) knots 0 0 0 0 1 1 1 1
  spline S252 degree 3 poles (1.5681, 12.9333) (2.0349, 13.2905) (2.4064, 13.5334) (2.4826, 13.5334) knots 0 0 0 0 1 1 1 1
  spline S253 degree 3 poles (2.4826, 13.5334) (2.5016, 13.5334) (2.5302, 13.5095) (2.5492, 13.4762) knots 0 0 0 0 1 1 1 1
  spline S254 degree 3 poles (2.5492, 13.4762) (2.5683, 13.4476) (2.5159, 13.3619) (2.4159, 13.2762) knots 0 0 0 0 1 1 1 1
  spline S255 degree 3 poles (2.4159, 13.2762) (2.2016, 13.0904) (1.3252, 12.4903) (1.0442, 12.3379) knots 0 0 0 0 1 1 1 1
  spline S256 degree 3 poles (1.0442, 12.3379) (0.9252, 12.276) (0.8014, 12.1951) (0.768, 12.1665) knots 0 0 0 0 1 1 1 1